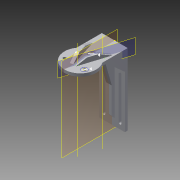
# Autodesk Inventor part: gimbal_yaw_brushless
Saved by Autodesk Inventor 2015 SP1 (Build 190203100, 203)
## iProperties
Created: 2015-08-06
Part Number: gimbal_yaw_brushless
Material: ABS Plastic
Document SubType Name: Modeling
Designer: Alexandre Cherpillod
Density: 1.06 g/cm^3
Appearance: Smooth - White
Mass: 4.03728 g
Surface Area: 41.4007 cm^2
Volume: 3.80876 cm^3
Author: Alexandre Cherpillod
Autodesk Inventor part; units mm, degrees
ref_plane "XZ Plane" through (0, 0, 0) normal (0, 1, 0) x (-1, 0, 0)
ref_plane "XY Plane" through (0, 0, 0) normal (0, 0, 1) x (1, 0, 0)
sketch "Sketch1" plane through (0, 0, 0) normal (0, 1, 0) x (-1, 0, 0)
  line L0 (-9, 40) -> (9, 40)
  line L1 (9, 40) -> (9, -9.6569)
  line L2 (9, -9.6569) -> (-9, -9.6569)
  line L3 (-9, -9.6569) -> (-9, 40)
  line L4 (-9, 40) -> (9, -9.6569) construction
  line L5 (9, 40) -> (-9, -9.6569) construction
  line L6 (0, -32.0453) -> (0, 52.0076) construction
  line L7 (-14.8076, 0) -> (25.8453, 0) construction
  line L8 (0, 0) -> (20.0378, -20.0378) construction
  line L9 (5.6569, -6.6569) -> (5.6569, 24.6569) construction
  line L10 (6.6569, -5.6569) -> (6.6569, 23.6569)
  line L11 (4.6569, 23.6569) -> (4.6569, -5.6569)
  arc A0 (4.6569, -5.6569) -> (6.6569, -5.6569) centre (5.6569, -5.6569) ccw
  arc A1 (6.6569, 23.6569) -> (4.6569, 23.6569) centre (5.6569, 23.6569) ccw
  line L12 (0, 0) -> (13.8345, 13.8345) construction
  line L13 (-5.6569, -6.6569) -> (-5.6569, 24.6569) construction
  line L14 (-6.6569, -5.6569) -> (-6.6569, 23.6569)
  line L15 (-4.6569, 23.6569) -> (-4.6569, -5.6569)
  arc A2 (-6.6569, -5.6569) -> (-4.6569, -5.6569) centre (-5.6569, -5.6569) ccw
  arc A3 (-4.6569, 23.6569) -> (-6.6569, 23.6569) centre (-5.6569, 23.6569) ccw
  point P0 (0, 15.1716)
  point P1 (0, 15.1716)
  point P2 (5.6569, -5.6569)
  point P3 (5.6569, 9)
  point P4 (5.6569, 5.6569)
  point P5 (-5.6569, -5.6569)
  point P6 (-5.6569, 9)
  point P7 (-5.6569, 5.6569)
  dimension "d34" = 18
  dimension "d35" = 45
  dimension "d36" = 8
  dimension "d37" = 2
  dimension "d38" = 0
  dimension "d40" = 45
  dimension "d41" = 18
  dimension "d42" = 4
  dimension "d43" = 40
  constraints: 32 end point, 13 point on line, 12 point on circle, 11 symmetric about line, 4 centre point, 4 midpoint, 4 tangent, 3 parallel, 1 horizontal, 1 perpendicular, 1 vertical, 2 other
  measures "d34" distance of L1.end L2.end
  measures "d35" angle of L6 L8
  measures "d36" distance of L8.start point (5.657, -5.657)
  measures "d37" diameter of A1
  measures "d38" distance of A0.centre point (5.657, -5.657)
  measures "d40" angle of L6 L12
  measures "d41" distance of A1.centre point (5.657, 5.657)
  measures "d42" distance from line of L2 A0.centre
  measures "d43" distance from line of L0 L8.start
extrude "Extrusion1" add sketch "Sketch1" against normal blind 2
sketch "Sketch4" plane through (-9, 0, 40) normal (0, 0, 1) x (1, 0, 0)
  line L0 (18, 0) -> (18, -2) construction
  line L1 (0, 0) -> (18, 0)
  line L2 (18, 0) -> (18, -17.6754)
  line L3 (9, -39.0627) -> (9, -2) construction
  line L4 (18, -2) -> (0, -2) construction
  line L5 (9, -24) -> (14.2107, -27.0084) construction
  circle A0 centre (15.9282, -28) radius 1
  circle A1 centre (9, -16) radius 1
  circle A2 centre (2.0718, -28) radius 1
  arc A3 (0, -17.6754) -> (18, -17.6754) centre (9, -24) ccw
  line L6 (0, -17.6754) -> (0, 0)
  point P0 (9, 0)
  dimension "d44" = 60
  dimension "d45" = 2
  dimension "d46" = 8
  dimension "d49" = 360
  dimension "d51" = 22
  dimension "d53" = 22
  constraints: 10 end point, 4 centre point, 2 point on circle, 2 point on line, 1 coincident, 1 horizontal, 1 midpoint, 1 parallel, 1 perpendicular, 1 vertical, 7 other
  measures "d44" angle of L3 L5
  measures "d45" diameter of A0
  measures "d46" distance of L5.start A0.centre
  measures "d51" distance from line of L4 L5.start
  measures "d53" diameter of A3
extrude "Extrusion4" add sketch "Sketch4" against normal blind 2
sketch "Sketch5" plane through (-9, -2, -9.6569) normal (-1, 0, 0) x (0, 0, 1)
  line L0 (47.6569, 0) -> (47.6569, -15.6754) projected
  line L1 (47.6569, -12.5494) -> (36.3362, 0)
  line L2 (47.6569, 0) -> (0, 0) projected
  line L3 (47.6569, 0) -> (47.6569, -12.5494)
  line L4 (47.6569, 0) -> (36.3362, 0)
  point P0 (9.6569, 2)
  constraints: 6 end point, 2 point on line, 1 collinear, 1 perpendicular
extrude "Extrusion5" add sketch "Sketch5" against normal blind 2
pattern_linear "Rectangular Pattern1" count 2 spacing 16 along (1, 0, 0) of "Extrusion5"
sketch "Sketch6" plane through (0, 0, 0) normal (1, 0, 0) x (0, 1, 0)
  line L0 (-14.5494, 38) -> (-2, 38) construction
  line L1 (-10.3568, 38) -> (-4.0789, 15.9865)
  line L2 (0, 40) -> (0, -9.6569) projected
  line L3 (-2, 38) -> (-10.3568, 38)
  line L4 (-4.0789, 15.9865) -> (-4.0789, -2.2693)
  line L5 (-4.0789, -2.2693) -> (-2, -4.6891)
  line L6 (-2, -4.6891) -> (-2, 38)
  point P0 (0, 0)
  constraints: 10 end point, 2 vertical, 1 collinear, 1 point on line
extrude "Extrusion6" add sketch "Sketch6" along normal mid plane 4
sketch "Sketch7" plane through (-9, 0, 40) normal (0, 0, 1) x (1, 0, 0)
  circle A0 centre (9, -16) radius 1 construction
  circle A1 centre (9, -16) radius 2 construction
  circle A2 centre (15.9282, -28) radius 1 construction
  circle A3 centre (15.9282, -28) radius 2 construction
  point P0 (9, 0)
  point P1 (14.689, -14.1786)
  point P2 (10.5252, -27.4837)
  dimension "d63" = 4
  dimension "d64" = 4
  constraints: 2 centre point, 2 coincident
  measures "d63" diameter of A1
  measures "d64" diameter of A3
ref_plane "Work Plane2" through (1.5252, -27.4837, 40) normal (-0.9544, 0.2987, 0) x (0, 0, 1)
sketch "Sketch8" plane through (1.5252, -27.4837, 40) normal (-0.9544, 0.2987, 0) x (0, 0, 1)
  line L0 (0, 11.593) -> (0, -8.1309) projected
  line L1 (0, -1.506) -> (3.29, 4.6767)
  line L2 (3.29, 4.6767) -> (3.29, 10.9801)
  line L3 (3.29, 10.9801) -> (0, 18.7943)
  line L4 (0, 23.0857) -> (0, 6.217) projected
  line L5 (0, -1.506) -> (0, 18.7943)
  point P0 (-40, 25.7737)
  constraints: 8 end point, 4 point on line, 1 collinear, 1 parallel
extrude "Extrusion7" add sketch "Sketch8" along normal mid plane 2
mirror "Mirror1" about plane through (0, 0, 0) normal (1, 0, 0) of "Extrusion7"
body "Solid1"
